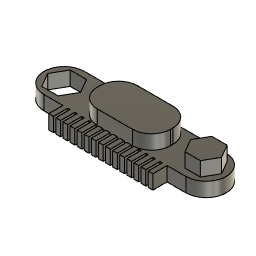
modularfingers v11 (Autodesk Fusion 360 design; units mm, degrees)
Autodesk Fusion 360 part; units mm, degrees
sketch "Sketch1" plane through (0, 0, 0) normal (0, 0, 1) x (1, 0, 0)
  line L0 (0, -4.25) -> (30, -4.25)
  arc A0 (30, -4.25) -> (30, 4.25) centre (30, 0) ccw
  line L1 (30, 4.25) -> (0, 4.25)
  arc A1 (0, 4.25) -> (0, -4.25) centre (0, 0) ccw
  line L2 (0, 0) -> (30, 0) construction
  circle A2 centre (0, 0) radius 3 construction
  line L3 (-1.7321, 3) -> (-3.4641, 0)
  line L4 (-3.4641, 0) -> (-1.7321, -3)
  line L5 (-1.7321, -3) -> (1.7321, -3)
  line L6 (1.7321, -3) -> (3.4641, 0)
  line L7 (3.4641, 0) -> (1.7321, 3)
  line L8 (1.7321, 3) -> (-1.7321, 3)
  circle A3 centre (30, 0) radius 2.825 construction
  line L9 (33.262, 0) -> (31.631, 2.825)
  line L10 (31.631, 2.825) -> (28.369, 2.825)
  line L11 (28.369, 2.825) -> (26.738, 0)
  line L12 (26.738, 0) -> (28.369, -2.825)
  line L13 (28.369, -2.825) -> (31.631, -2.825)
  line L14 (31.631, -2.825) -> (33.262, 0)
  line L15 (18.738, -4.25) -> (11.262, -4.25)
  line L16 (7.262, -0.25) -> (7.262, 0.25)
  line L17 (11.262, 4.25) -> (18.738, 4.25)
  line L18 (22.738, 0.25) -> (22.738, -0.25)
  line L19 (22.738, -4.25) -> (7.262, 4.25) construction
  line L20 (7.262, -4.25) -> (22.738, 4.25) construction
  arc A4 (11.262, 4.25) -> (7.262, 0.25) centre (11.262, 0.25) ccw
  arc A5 (7.262, -0.25) -> (11.262, -4.25) centre (11.262, -0.25) ccw
  arc A6 (18.738, -4.25) -> (22.738, -0.25) centre (18.738, -0.25) ccw
  arc A7 (22.738, 0.25) -> (18.738, 4.25) centre (18.738, 0.25) ccw
  point P0 (30, 0)
  point P1 (15, 0)
  dimension "d1" = 30
  dimension "d2" = 4.25
  dimension "d14" = 60
  dimension "d15" = 5.65
  dimension "d16" = 6
  dimension "d17" = 60
  dimension "d18" = 4
  dimension "d19" = 4
  constraint tangent L0 A0
  constraint tangent A0 L1
  constraint parallel L0 L1
  constraint tangent L1 A1
  constraint tangent L0 A1
  constraint horizontal L2
  constraint coincident A1.centre L2.start
  constraint concentric A1 A2
  constraint concentric A0 A3
  constraint coincident P0 A0.centre
  constraint tangent A3 L9
  constraint tangent A2 L7
  constraint horizontal L15
  constraint perpendicular L15 L16
  constraint parallel L15 L17
  constraint parallel L16 L18
  constraint coincident L19 P1
  constraint coincident L20 P1
  constraint coincident L0 L19.start
  constraint midpoint L2 P1
  constraint coincident L19.end L16
  constraint coincident L19.end L17
  constraint tangent L16 A4
  constraint tangent L17 A4
  constraint coincident L20.start L16
  constraint coincident L20.start L15
  constraint tangent L16 A5
  constraint tangent L15 A5
  constraint equal A4 A5
  constraint coincident L19.start L18
  constraint coincident L19.start L15
  constraint tangent L18 A6
  constraint tangent L15 A6
  constraint equal A4 A6
  constraint coincident L20.end L18
  constraint coincident L20.end L17
  constraint tangent L18 A7
  constraint tangent L17 A7
  constraint equal A4 A7
  measures "d1" distance of A0.end L1.end
  measures "d2" radius of A0
  measures "d14" angle of L2 L7
  measures "d15" diameter of A3
  measures "d16" diameter of A2
  measures "d17" angle of L2 L14
  measures "d18" distance of L11.end L18
  measures "d19" radius of A4
extrude "Extrude1" add sketch "Sketch1" along normal blind 3 contours L0 L1 A1 L16 A4 A5 | L0 A0 L1 L18 A6 A7 makes body 1 at (4.2732, -1.6372, 0) makes body 2 at (25.8943, 1.4006, 0)
extrude "Extrude3" add sketch "Sketch1" along normal blind 6 contours L0 L1 L15 L16 L17 L18 A4 A5 A6 A7 | L9 L10 L11 L12 L13 L14 bodies 1 2
sketch "Sketch3" plane through (0, -4.25, 0) normal (0, -1, 0) x (1, 0, 0)
  line L0 (0, 0) -> (30, 0)
  line L1 (30, 0) -> (30, 3)
  line L2 (30, 3) -> (18.738, 3)
  line L3 (18.738, 3) -> (18.738, 6)
  line L4 (18.738, 6) -> (11.262, 6)
  line L5 (11.262, 6) -> (11.262, 3)
  line L6 (11.262, 3) -> (0, 3)
  line L7 (0, 3) -> (0, 0)
  line L8 (4, 3) -> (5, 3)
  line L9 (5, 3) -> (5, 0)
  line L10 (5, 0) -> (4, 0)
  line L11 (4, 0) -> (4, 3)
  line L12 (6.5, 3) -> (6.5, 0)
  line L13 (5.5, 3) -> (6.5, 3)
  line L14 (5.5, 0) -> (5.5, 3)
  line L15 (6.5, 0) -> (5.5, 0)
  line L16 (8, 3) -> (8, 0)
  line L17 (7, 3) -> (8, 3)
  line L18 (7, 0) -> (7, 3)
  line L19 (8, 0) -> (7, 0)
  line L20 (9.5, 3) -> (9.5, 0)
  line L21 (8.5, 3) -> (9.5, 3)
  line L22 (8.5, 0) -> (8.5, 3)
  line L23 (9.5, 0) -> (8.5, 0)
  line L24 (11, 3) -> (11, 0)
  line L25 (10, 3) -> (11, 3)
  line L26 (10, 0) -> (10, 3)
  line L27 (11, 0) -> (10, 0)
  line L28 (12.5, 3) -> (12.5, 0)
  line L29 (11.5, 3) -> (12.5, 3)
  line L30 (11.5, 0) -> (11.5, 3)
  line L31 (12.5, 0) -> (11.5, 0)
  line L32 (14, 3) -> (14, 0)
  line L33 (13, 3) -> (14, 3)
  line L34 (13, 0) -> (13, 3)
  line L35 (14, 0) -> (13, 0)
  line L36 (15.5, 3) -> (15.5, 0)
  line L37 (14.5, 3) -> (15.5, 3)
  line L38 (14.5, 0) -> (14.5, 3)
  line L39 (15.5, 0) -> (14.5, 0)
  line L40 (17, 3) -> (17, 0)
  line L41 (16, 3) -> (17, 3)
  line L42 (16, 0) -> (16, 3)
  line L43 (17, 0) -> (16, 0)
  line L44 (18.5, 3) -> (18.5, 0)
  line L45 (17.5, 3) -> (18.5, 3)
  line L46 (17.5, 0) -> (17.5, 3)
  line L47 (18.5, 0) -> (17.5, 0)
  line L48 (20, 3) -> (20, 0)
  line L49 (19, 3) -> (20, 3)
  line L50 (19, 0) -> (19, 3)
  line L51 (20, 0) -> (19, 0)
  line L52 (21.5, 3) -> (21.5, 0)
  line L53 (20.5, 3) -> (21.5, 3)
  line L54 (20.5, 0) -> (20.5, 3)
  line L55 (21.5, 0) -> (20.5, 0)
  line L56 (23, 3) -> (23, 0)
  line L57 (22, 3) -> (23, 3)
  line L58 (22, 0) -> (22, 3)
  line L59 (23, 0) -> (22, 0)
  line L60 (24.5, 3) -> (24.5, 0)
  line L61 (23.5, 3) -> (24.5, 3)
  line L62 (23.5, 0) -> (23.5, 3)
  line L63 (24.5, 0) -> (23.5, 0)
  line L64 (26, 3) -> (26, 0)
  line L65 (25, 3) -> (26, 3)
  line L66 (25, 0) -> (25, 3)
  line L67 (26, 0) -> (25, 0)
  dimension "d39" = 1
  dimension "d40" = 4
  dimension "d47" = 21
  dimension "d48" = 0
  constraint horizontal L8
  constraint vertical L9
  constraint horizontal L10
  constraint vertical L11
  constraint coincident L0 L9.end
  constraint coincident L6 L8.start
  measures "d39" distance of L9.end L10.end
  measures "d40" distance of L7 L11
extrude "Extrude5" add sketch "Sketch3" along normal blind 3 contours L0 L6 L8 L9 L10 L11 | L0 L6 L12 L13 L14 L15 | L0 L6 L16 L17 L18 L19 | L0 L6 L20 L21 L22 L23 | L0 L6 L24 L25 L26 L27 | L0 L28 L29 L30 L31 | L0 L32 L33 L34 L35 | L0 L36 L37 L38 L39 | L0 L2 L48 L49 L50 L51 | L0 L40 L41 L42 L43 | L0 L2 L52 L53 L54 L55 | L0 L44 L45 L46 L47 | L0 L2 L56 L57 L58 L59 | L0 L2 L60 L61 L62 L63 | L0 L2 L64 L65 L66 L67 bodies 1
equation "d1 = length"
equation "d2 = arc_Length"
equation "height = 6 mm"
equation "length = 30 mm"
equation "total_length = 30 mm + 8.5 mm"
equation "arc_Length = ( total_length - length ) / 2"
equation "DegreePolygon = ( 360 / 6 ) * 1 deg"
equation "Polygon_Length = 6 mm"
equation "NPolygonSides = 6"
equation "d14 = DegreePolygon"
equation "d15 = Polygon_Length - Hole_OFFSET"
equation "d16 = Polygon_Length"
equation "d17 = DegreePolygon"
equation "d18 = offsetdistance"
equation "d19 = arc_Polygon"
equation "arc_Polygon = 4 mm"
equation "offsetdistance = 4 mm"
equation "d22 = ( height / 2 mm ) * 1 mm"
equation "d26 = height"
equation "Hole_OFFSET = 0.35 mm"
equation "d39 = pattounes_width"
equation "d40 = pattounes_offset"
equation "pattounes_offset = 4 mm"
equation "pattounes_width = 1 mm"
equation "NPattounes = 15"
equation "d45 = NPattounes"
equation "d47 = length - pattounes_offset * 2 - pattounes_width"
